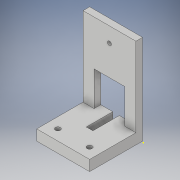
# Autodesk Inventor part: End Frame 2
Saved by Autodesk Inventor 2017 (Build 210142000, 142)
## iProperties
Created: 2018-03-09
Part Number: End Frame 2
Material: Generic
Document SubType Name: Modeling
Designer: Russ
Density: 1 g/cm^3
Appearance: Default
Author: Russ
Autodesk Inventor part; units mm, degrees
ref_plane "YZ Plane" through (0, 0, 0) normal (1, 0, 0) x (0, 1, 0)
ref_plane "XZ Plane" through (0, 0, 0) normal (0, 1, 0) x (-1, 0, 0)
ref_plane "XY Plane" through (0, 0, 0) normal (0, 0, 1) x (1, 0, 0)
sketch "Sketch1" plane through (0, 0, 0) normal (0, 0, 1) x (1, 0, 0)
  line L0 (-51.5087, 0.9312) -> (-0.7087, 0.9312)
  line L1 (-0.7087, 0.9312) -> (-0.7087, 11.0912)
  line L2 (-0.7087, 11.0912) -> (-51.5087, 11.0912)
  line L3 (-51.5087, 11.0912) -> (-51.5087, 0.9312)
  dimension "d1" = 10.16
  dimension "d2" = 50.8
  constraints: 8 end point, 2 parallel, 1 horizontal, 1 perpendicular
  measures "d1" distance of L0.end L1.end
  measures "d2" distance of L0.start L0.end
extrude "Extrusion1" add sketch "Sketch1" along normal blind 50.8
sketch "Sketch2" plane through (0, 0, 0) normal (0, 0, -1) x (-1, 0, 0)
  arc A0 (43.6087, 20.9733) -> (43.6087, 27.9733) centre (43.6087, 24.4733) ccw
  line L0 (8.6087, 27.9733) -> (12.5532, 27.9733)
  line L1 (8.6087, 27.9733) -> (12.5532, 27.9733)
  line L2 (8.6087, 20.9733) -> (12.5532, 20.9733)
  line L3 (8.6087, 20.9733) -> (12.5532, 20.9733)
  arc A1 (9.0398, 27.9733) -> (9.0398, 20.9733) centre (8.6512, 24.4733) ccw
  line L4 (43.6087, 27.9733) -> (39.6641, 27.9733)
  line L5 (39.6641, 27.9733) -> (43.6087, 27.9733)
  line L6 (43.6087, 20.9733) -> (39.6641, 20.9733)
  line L7 (39.6641, 20.9733) -> (43.6087, 20.9733)
  arc A2 (18.8087, 11.9789) -> (18.362, 12.8118) centre (17.8087, 11.9789) ccw
  line L8 (18.8087, 8.6771) -> (18.8087, 11.5509)
  line L9 (18.8087, 11.9789) -> (18.8087, 8.6771)
  line L10 (18.8087, 8.6771) -> (18.8087, 7.6771)
  arc A3 (18.8087, 8.6771) -> (19.8087, 7.6771) centre (19.8087, 8.6771) ccw
  line L11 (18.8087, 7.6771) -> (33.4087, 7.6771)
  line L12 (33.4087, 11.9789) -> (33.4087, 11.5509)
  line L13 (33.4087, 7.6771) -> (33.4087, 11.9789)
  arc A4 (33.8554, 12.8118) -> (33.4087, 11.9789) centre (34.4087, 11.9789) ccw
  arc A5 (33.4087, 11.9789) -> (33.4087, 11.9789) centre (34.4087, 11.9789) ccw
  arc A6 (18.8087, 11.9789) -> (18.362, 12.8118) centre (17.8087, 11.9789) ccw
  arc A7 (12.5532, 20.9733) -> (18.362, 12.8118) centre (26.1087, 24.4733) ccw
  arc A8 (33.8554, 12.8118) -> (39.6641, 20.9733) centre (26.1087, 24.4733) ccw
  arc A9 (39.6641, 27.9733) -> (12.5532, 27.9733) centre (26.1087, 24.4733) ccw
  line L14 (0.7087, 11.0912) -> (51.5087, 11.0912) projected
  circle A10 centre (26.1087, 24.4733) radius 14
  line L15 (0.7087, 0.9312) -> (0.7087, 11.0912) projected
  line L16 (0.7087, 11.0912) -> (51.5087, 11.0912)
  line L17 (51.5087, 11.0912) -> (51.5087, 61.8912)
  line L18 (51.5087, 61.8912) -> (0.7087, 61.8912)
  line L19 (0.7087, 61.8912) -> (0.7087, 11.0912)
  line L20 (11.3767, 28.2833) -> (11.3767, 11.0912)
  line L21 (11.3767, 28.2833) -> (11.3767, 44.1112)
  line L22 (11.3767, 44.1112) -> (40.8407, 44.1112)
  line L23 (40.8407, 44.1112) -> (40.8407, 11.0912)
  point P0 (0, 0)
  point P1 (26.1087, 11.0912)
  dimension "d6" = 0
  dimension "d7" = 50.8
  dimension "d9" = 14.732
  dimension "d10" = 14.732
  dimension "d11" = 33.02
  constraints: 44 end point, 19 point on circle, 10 centre point, 6 collinear, 6 point on line, 4 perpendicular, 2 coincident, 2 concentric, 2 horizontal, 2 parallel, 2 tangent, 1 horizontal alignment, 1 midpoint, 3 other
  measures "d6" horizontal distance of A7.centre point (26.109, 11.091)
  measures "d7" distance of L16.end L17.end
  measures "d9" distance from line of point (26.109, 11.091) L20
  measures "d10" distance from line of L23 point (26.109, 11.091)
  measures "d11" distance of L22.end L23.end
extrude "Extrusion2" add sketch "Sketch2" against normal blind 6.35 contours L6 L23 L4 A0 | A0 L4 L23 L22 L21 L20 L0 A1 L2 L14 L19 L18 L17 L6 | L20 L2 A1 L0
sketch "Sketch3" plane through (0, 0, 0) normal (0, 0, -1) x (-1, 0, 0)
  arc A0 (43.6087, 24.541) -> (43.6087, 31.541) centre (43.6087, 28.041) ccw
  line L0 (8.6087, 31.541) -> (12.5532, 31.541)
  line L1 (8.6087, 31.541) -> (12.5532, 31.541)
  line L2 (8.6087, 24.541) -> (12.5532, 24.541)
  line L3 (8.6087, 24.541) -> (12.5532, 24.541)
  arc A1 (9.0398, 31.541) -> (9.0398, 24.541) centre (8.6512, 28.041) ccw
  line L4 (43.6087, 31.541) -> (39.6641, 31.541)
  line L5 (39.6641, 31.541) -> (43.6087, 31.541)
  line L6 (43.6087, 24.541) -> (39.6641, 24.541)
  line L7 (39.6641, 24.541) -> (43.6087, 24.541)
  arc A2 (18.8087, 15.5466) -> (18.362, 16.3795) centre (17.8087, 15.5466) ccw
  line L8 (18.8087, 12.2448) -> (18.8087, 15.1185)
  line L9 (18.8087, 15.5466) -> (18.8087, 12.2448)
  line L10 (18.8087, 12.2448) -> (18.8087, 11.2448)
  arc A3 (18.8087, 12.2448) -> (19.8087, 11.2448) centre (19.8087, 12.2448) ccw
  line L11 (18.8087, 11.2448) -> (33.4087, 11.2448)
  line L12 (33.4087, 15.5466) -> (33.4087, 15.1185)
  line L13 (33.4087, 11.2448) -> (33.4087, 15.5466)
  arc A4 (33.8554, 16.3795) -> (33.4087, 15.5466) centre (34.4087, 15.5466) ccw
  arc A5 (33.4087, 15.5466) -> (33.4087, 15.5466) centre (34.4087, 15.5466) ccw
  arc A6 (18.8087, 15.5466) -> (18.362, 16.3795) centre (17.8087, 15.5466) ccw
  arc A7 (12.5532, 24.541) -> (18.362, 16.3795) centre (26.1087, 28.041) ccw
  arc A8 (33.8554, 16.3795) -> (39.6641, 24.541) centre (26.1087, 28.041) ccw
  arc A9 (39.6641, 31.541) -> (12.5532, 31.541) centre (26.1087, 28.041) ccw
  line L14 (11.3767, 11.0912) -> (40.8407, 11.0912) projected
  circle A10 centre (26.1087, 28.041) radius 25.7175
  circle A11 centre (26.1087, 61.7236) radius 7.62
  line L15 (0.7087, 61.8912) -> (51.5087, 61.8912) projected
  line L16 (0.7087, 0.9312) -> (0.7087, 61.8912) projected
  line L17 (0.7087, 61.8912) -> (51.5087, 61.8912)
  line L18 (51.5087, 61.8912) -> (51.5087, 76.3692)
  line L19 (51.5087, 76.3692) -> (0.7087, 76.3692)
  line L20 (0.7087, 76.3692) -> (0.7087, 61.8912)
  point P0 (0, 0)
  point P1 (26.1087, 11.0912)
  point P2 (26.1087, 61.8912)
  dimension "d15" = 0
  dimension "d16" = 51.435
  dimension "d17" = 15.24
  dimension "d18" = 0
  dimension "d19" = 14.478
  constraints: 36 end point, 19 point on circle, 11 centre point, 6 collinear, 3 point on line, 2 coincident, 2 midpoint, 2 parallel, 2 perpendicular, 2 tangent, 1 concentric, 1 horizontal, 1 horizontal alignment, 3 other
  measures "d15" horizontal distance of point (26.109, 11.091) point (26.109, 28.041)
  measures "d16" diameter of A10
  measures "d17" diameter of A11
  measures "d18" horizontal distance of point (26.109, 61.891) A11.centre
  measures "d19" distance of L17.end L18.end
extrude "Extrusion3" add sketch "Sketch3" against normal blind 6.35 contours L20 L19 L18 L15 A11 | A11 L15 picked at (24.5986, 64.5356)
sketch "Sketch5" plane through (0, 0, 0) normal (0, 0, -1) x (-1, 0, 0)
  line L0 (0.7087, 11.0912) -> (51.5087, 11.0912) projected
  line L1 (26.1087, 11.0912) -> (26.1087, 35.6872)
  line L2 (26.1087, 35.6872) -> (26.1087, 61.4047)
  circle A0 centre (26.1087, 72.7077) radius 7.62
  circle A1 centre (26.1087, 72.7077) radius 1.905
  line L3 (0.7087, 76.3692) -> (51.5087, 76.3692) projected
  point P0 (0, 0)
  dimension "d26" = 24.596
  dimension "d27" = 25.7175
  dimension "d28" = 15.24
  dimension "d29" = 11.303
  dimension "d30" = 3.81
  constraints: 4 end point, 2 centre point, 2 vertical, 1 coincident, 1 midpoint
  measures "d26" distance of L1.start L1.end
  measures "d27" distance of L1.end L2.end
  measures "d28" diameter of A0
  measures "d29" distance of L2.end A0.centre
  measures "d30" diameter of A1
extrude "Extrusion5" cut sketch "Sketch5" against normal up to next contours A1
sketch "Sketch6" plane through (0, 0, 0) normal (0, 0, -1) x (-1, 0, 0)
  line L0 (0.7087, 76.3692) -> (51.5087, 76.3692) projected
  line L1 (0.7087, 76.3692) -> (51.5087, 76.3692)
  line L2 (51.5087, 76.3692) -> (51.5087, 87.1857)
  line L3 (51.5087, 87.1857) -> (0.7087, 87.1857)
  line L4 (0.7087, 87.1857) -> (0.7087, 76.3692)
  circle A0 centre (26.1087, 72.7077) radius 1.905 projected
  point P0 (0, 0)
  dimension "d33" = 14.478
  constraints: 8 end point, 2 parallel, 1 horizontal, 1 perpendicular
  measures "d33" distance from line of A0.centre L3
extrude "Extrusion6" add sketch "Sketch6" against normal blind 6.35 contours L4 L3 L2 L0
sketch "Sketch8" plane through (-51.5087, 11.0912, 50.8) normal (0, 1, 0) x (1, 0, 0)
  circle A0 centre (40.64, 10.16) radius 2.3813
  circle A1 centre (10.16, 10.16) radius 2.3813
  line L0 (50.8, 0) -> (0, 0) projected
  line L1 (50.8, 50.8) -> (50.8, 0) projected
  line L2 (0, 44.45) -> (0, 0) projected
  point P0 (51.5087, 50.8)
  dimension "d36" = 4.7625
  dimension "d37" = 4.7625
  dimension "d38" = 10.16
  dimension "d39" = 10.16
  dimension "d40" = 10.16
  dimension "d41" = 10.16
  constraints: 2 centre point
  measures "d36" diameter of A1
  measures "d37" diameter of A0
  measures "d38" distance from line of L0 A0.centre
  measures "d39" distance from line of L1 A0.centre
  measures "d40" distance from line of L0 A1.centre
  measures "d41" distance from line of L2 A1.centre
extrude "Extrusion7" cut sketch "Sketch8" against normal up to next
sketch "Sketch9" plane through (0, 0, 0) normal (0, 0, -1) x (-1, 0, 0)
  line L0 (11.3767, 11.0912) -> (40.8407, 11.0912) projected
  line L1 (26.1087, 11.0912) -> (26.1087, 0.9312)
  line L2 (51.5087, 0.9312) -> (0.7087, 0.9312) projected
  line L3 (22.9337, 11.0912) -> (29.2837, 11.0912)
  line L4 (29.2837, 11.0912) -> (29.2837, 0.9312)
  line L5 (29.2837, 0.9312) -> (22.9337, 0.9312)
  line L6 (22.9337, 0.9312) -> (22.9337, 11.0912)
  point P0 (0, 0)
  dimension "d45" = 6.35
  dimension "d46" = 3.175
  constraints: 10 end point, 2 midpoint, 2 parallel, 2 point on line, 1 horizontal, 1 perpendicular
  measures "d45" distance between parallel lines of L4 L6
  measures "d46" distance between parallel lines of L4 L1
extrude "Extrusion8" cut sketch "Sketch9" against normal blind 25.4
sketch "Sketch10" plane through (0, 0, 0) normal (0, 0, -1) x (-1, 0, 0)
  point P0 (0, 0)
body "Solid1"
